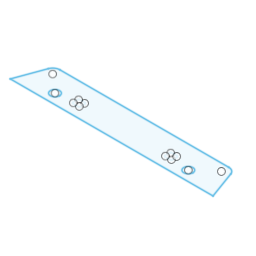
Zaagblad_C (Autodesk Fusion 360 archive; units mm, degrees)
design "Zaagblad_C" references "autodesk generic router xyz", "autodesk generic router xyz"
Autodesk Fusion 360 part; units mm, degrees
sketch "C_omtrek" plane through (0, 0, 0) normal (0, 0, 1) x (1, 0, 0)
  line L0 (0, -881.7664) -> (1220, -881.7664)
  line L1 (1220, -881.7664) -> (1220, -1491.7664)
  line L2 (1220, -1491.7664) -> (0, -1491.7664)
  line L3 (0, -1491.7664) -> (0, -881.7664)
  dimension "d47" = 610
  constraint horizontal L0
  constraint vertical L1
  constraint horizontal L2
  constraint vertical L3
  measures "d47" distance of L0.start L2.end
sketch "C_middle_holes" plane through (0, 0, 0) normal (0, 0, 1) x (1, 0, 0)
  line L0 (45, -1471.7664) -> (895, -1471.7664)
  line L1 (920, -1446.7664) -> (920, -926.7664)
  line L2 (895, -901.7664) -> (45, -901.7664)
  line L3 (20, -926.7664) -> (20, -1446.7664)
  arc A0 (20, -1446.7664) -> (45, -1471.7664) centre (45, -1446.7664) ccw
  arc A1 (45, -901.7664) -> (20, -926.7664) centre (45, -926.7664) ccw
  arc A2 (920, -926.7664) -> (895, -901.7664) centre (895, -926.7664) ccw
  arc A3 (895, -1471.7664) -> (920, -1446.7664) centre (895, -1446.7664) ccw
  line L4 (360, -1144.2664) -> (580, -1144.2664)
  line L5 (580, -1144.2664) -> (580, -1214.2664)
  line L6 (580, -1214.2664) -> (360, -1214.2664)
  line L7 (360, -1214.2664) -> (360, -1144.2664)
  line L8 (350, -1134.2664) -> (590, -1134.2664)
  line L9 (590, -1134.2664) -> (590, -1224.2664)
  line L10 (590, -1224.2664) -> (350, -1224.2664)
  line L11 (350, -1224.2664) -> (350, -1134.2664)
  circle A4 centre (280, -1179.2664) radius 48.25
  circle A5 centre (660, -1179.2664) radius 48.25
  line L12 (470, -1224.2664) -> (470, -1550) construction
  point P0 (20, -1471.7664)
  point P1 (920, -1471.7664)
  point P2 (20, -901.7664)
  dimension "d50" = 900
  dimension "d51" = 570
  dimension "d52" = 25
  dimension "d53" = 25
  dimension "d54" = 25
  dimension "d55" = 25
  dimension "d195" = -10
  dimension "d196" = 96.5
  dimension "d197" = 96.5
  constraint horizontal L0
  constraint vertical L1
  constraint horizontal L2
  constraint vertical L3
  constraint coincident P0 L0
  constraint coincident P0 L3
  constraint tangent L0 A0
  constraint tangent L3 A0
  constraint coincident P2 L2
  constraint coincident P2 L3
  constraint tangent L2 A1
  constraint tangent L3 A1
  constraint tangent L1 A2
  constraint tangent L2 A2
  constraint coincident P1 L0
  constraint coincident P1 L1
  constraint tangent L0 A3
  constraint tangent L1 A3
  constraint midpoint L10 L12.start
  constraint perpendicular L10 L12
  measures "d50" distance of P0 P1
  measures "d51" distance of P0 P2
  measures "d52" radius of A0
  measures "d53" radius of A1
  measures "d54" radius of A2
  measures "d55" radius of A3
  measures "d196" diameter of A4
  measures "d197" diameter of A5
extrude "Extrude1" add sketch "C_omtrek" along normal blind 18
sketch "C_bottom_edge" plane through (0, 0, 0) normal (0, 0, 1) x (1, 0, 0)
  line L0 (178.8438, -1361.7664) -> (743.8334, -1361.7664)
  line L1 (155.3514, -1378.2159) -> (121.3018, -1471.7664)
  arc A0 (178.8438, -1361.7664) -> (155.3514, -1378.2159) centre (178.8438, -1386.7664) ccw
  arc A1 (767.3257, -1378.2159) -> (743.8334, -1361.7664) centre (743.8334, -1386.7664) ccw
  line L2 (767.3257, -1378.2159) -> (801.3753, -1471.7664)
  line L3 (121.3018, -1471.7664) -> (801.3753, -1471.7664)
  dimension "d188" = 25
  dimension "d177" = 25
  dimension "d178" = 25
  constraint horizontal L0
  constraint tangent L1 A0
  constraint tangent L0 A0
  constraint tangent A1 L2
  constraint tangent L0 A1
  measures "d177" radius of A0
  measures "d178" radius of A1
sketch "C_bottom_holes" plane through (0, 0, 0) normal (0, 0, 1) x (1, 0, 0)
  circle A0 centre (246.75, -1438.2664) radius 15
  circle A1 centre (693.25, -1438.2664) radius 15
  line L0 (305.75, -1415.6268) -> (325.75, -1415.6268)
  line L1 (328.25, -1418.1268) -> (328.25, -1435.918)
  line L2 (325.75, -1438.418) -> (305.75, -1438.418)
  line L3 (303.25, -1435.918) -> (303.25, -1418.1268)
  arc A2 (328.25, -1418.1268) -> (325.75, -1415.6268) centre (325.75, -1418.1268) ccw
  arc A3 (305.75, -1415.6268) -> (303.25, -1418.1268) centre (305.75, -1418.1268) ccw
  arc A4 (303.25, -1435.918) -> (305.75, -1438.418) centre (305.75, -1435.918) ccw
  arc A5 (325.75, -1438.418) -> (328.25, -1435.918) centre (325.75, -1435.918) ccw
  arc A6 (634.25, -1438.418) -> (636.75, -1435.918) centre (634.25, -1435.918) ccw
  arc A7 (611.75, -1435.918) -> (614.25, -1438.418) centre (614.25, -1435.918) ccw
  arc A8 (636.75, -1418.1268) -> (634.25, -1415.6268) centre (634.25, -1418.1268) ccw
  arc A9 (614.25, -1415.6268) -> (611.75, -1418.1268) centre (614.25, -1418.1268) ccw
  line L4 (614.25, -1415.6268) -> (634.25, -1415.6268)
  line L5 (611.75, -1435.918) -> (611.75, -1418.1268)
  line L6 (634.25, -1438.418) -> (614.25, -1438.418)
  line L7 (636.75, -1418.1268) -> (636.75, -1435.918)
  point P0 (660, -1179.2664)
  point P1 (303.25, -1415.6268)
  point P2 (328.25, -1415.6268)
  point P3 (636.75, -1415.6268)
  point P4 (611.75, -1415.6268)
  dimension "d206" = 30
  dimension "d207" = 30
  dimension "d208" = 25
  dimension "d210" = 2.5
  dimension "d211" = 2.5
  dimension "d212" = 2.5
  dimension "d213" = 2.5
  dimension "d214" = 25
  dimension "d215" = 2.5
  dimension "d216" = 2.5
  dimension "d217" = 2.5
  dimension "d218" = 2.5
  constraint horizontal L0
  constraint vertical L1
  constraint horizontal L2
  constraint vertical L3
  constraint coincident P2 L0
  constraint coincident P2 L1
  constraint tangent L0 A2
  constraint tangent L1 A2
  constraint coincident P1 L0
  constraint coincident P1 L3
  constraint tangent L0 A3
  constraint tangent L3 A3
  constraint tangent L2 A4
  constraint tangent L3 A4
  constraint tangent L1 A5
  constraint tangent L2 A5
  constraint horizontal L4
  constraint vertical L7
  constraint horizontal L6
  constraint vertical L5
  constraint coincident P3 L4
  constraint coincident P3 L7
  constraint tangent A8 L4
  constraint tangent A8 L7
  constraint coincident P4 L4
  constraint coincident P4 L5
  constraint tangent A9 L4
  constraint tangent A9 L5
  constraint tangent A7 L6
  constraint tangent A7 L5
  constraint tangent A6 L7
  constraint tangent A6 L6
  measures "d206" diameter of A0
  measures "d207" diameter of A1
  measures "d208" distance of P1 P2
  measures "d210" radius of A2
  measures "d211" radius of A3
  measures "d212" radius of A4
  measures "d213" radius of A5
  measures "d214" distance of P3 P4
  measures "d215" radius of A8
  measures "d216" radius of A9
  measures "d217" radius of A7
  measures "d218" radius of A6
sketch "Lasercutter_3mm" plane through (0, 0, 0) normal (0, 0, 1) x (1, 0, 0)
  line L0 (580, -1144.2664) -> (580, -1214.2664)
  line L1 (895, -901.7664) -> (45, -901.7664)
  arc A0 (895, -1471.7664) -> (920, -1446.7664) centre (895, -1446.7664) ccw
  arc A1 (920, -926.7664) -> (895, -901.7664) centre (895, -926.7664) ccw
  circle A2 centre (660, -1179.2664) radius 48.25
  line L2 (360, -1144.2664) -> (580, -1144.2664)
  line L3 (920, -1446.7664) -> (920, -926.7664)
  line L4 (20, -926.7664) -> (20, -1446.7664)
  arc A3 (45, -901.7664) -> (20, -926.7664) centre (45, -926.7664) ccw
  line L5 (580, -1214.2664) -> (360, -1214.2664)
  arc A4 (20, -1446.7664) -> (45, -1471.7664) centre (45, -1446.7664) ccw
  circle A5 centre (280, -1179.2664) radius 48.25
  line L6 (360, -1214.2664) -> (360, -1144.2664)
  point P0 (660, -1179.2664)
  dimension "d219" = -10
  dimension "d222" = 25
  dimension "d223" = 25
  dimension "d224" = 25
  dimension "d225" = 25
  dimension "d226" = 96.5
  dimension "d227" = 96.5
  constraint vertical L3
  constraint horizontal L1
  constraint vertical L4
  constraint tangent L4 A4
  constraint tangent L1 A3
  constraint tangent L4 A3
  constraint tangent A1 L3
  constraint tangent L1 A1
  constraint tangent A0 L3
  measures "d222" radius of A4
  measures "d223" radius of A3
  measures "d224" radius of A1
  measures "d225" radius of A0
  measures "d226" diameter of A5
  measures "d227" diameter of A2
sketch "Lasercutter_5mm" plane through (0, 0, 0) normal (0, 0, 1) x (1, 0, 0)
  line L0 (636.75, -1418.1268) -> (636.75, -1435.918)
  line L1 (611.75, -1435.918) -> (611.75, -1418.1268)
  arc A0 (611.75, -1435.918) -> (614.25, -1438.418) centre (614.25, -1435.918) ccw
  arc A1 (614.25, -1415.6268) -> (611.75, -1418.1268) centre (614.25, -1418.1268) ccw
  line L2 (328.25, -1418.1268) -> (328.25, -1435.918)
  line L3 (303.25, -1435.918) -> (303.25, -1418.1268)
  arc A2 (303.25, -1435.918) -> (305.75, -1438.418) centre (305.75, -1435.918) ccw
  arc A3 (305.75, -1415.6268) -> (303.25, -1418.1268) centre (305.75, -1418.1268) ccw
  circle A4 centre (246.75, -1438.2664) radius 15
  arc A5 (636.75, -1418.1268) -> (634.25, -1415.6268) centre (634.25, -1418.1268) ccw
  line L4 (325.75, -1438.418) -> (305.75, -1438.418)
  arc A6 (634.25, -1438.418) -> (636.75, -1435.918) centre (634.25, -1435.918) ccw
  line L5 (614.25, -1415.6268) -> (634.25, -1415.6268)
  line L6 (130.4954, -1471.7664) -> (809.5046, -1471.7664)
  line L7 (634.25, -1438.418) -> (614.25, -1438.418)
  circle A7 centre (693.25, -1438.2664) radius 15
  arc A8 (328.25, -1418.1268) -> (325.75, -1415.6268) centre (325.75, -1418.1268) ccw
  arc A9 (325.75, -1438.418) -> (328.25, -1435.918) centre (325.75, -1435.918) ccw
  line L8 (305.75, -1415.6268) -> (325.75, -1415.6268)
  arc A10 (775.5173, -1378.3869) -> (752.4948, -1362.2664) centre (752.4948, -1386.7664) ccw
  line L9 (187.5052, -1362.2664) -> (752.4948, -1362.2664)
  arc A11 (187.5052, -1362.2664) -> (164.4827, -1378.3869) centre (187.5052, -1386.7664) ccw
  line L10 (164.4827, -1378.3869) -> (130.4954, -1471.7664)
  line L11 (775.5173, -1378.3869) -> (809.5046, -1471.7664)
  dimension "d252" = 30
  dimension "d253" = 30
  dimension "d255" = 2.5
  dimension "d256" = 2.5
  dimension "d257" = 2.5
  dimension "d258" = 2.5
  dimension "d260" = 2.5
  dimension "d261" = 2.5
  dimension "d262" = 2.5
  dimension "d263" = 2.5
  constraint horizontal L6
  constraint horizontal L8
  constraint vertical L2
  constraint horizontal L4
  constraint vertical L3
  constraint tangent A8 L8
  constraint tangent L2 A8
  constraint tangent A3 L8
  constraint tangent L3 A3
  constraint tangent A2 L4
  constraint tangent L3 A2
  constraint tangent L2 A9
  constraint tangent L4 A9
  constraint horizontal L5
  constraint vertical L0
  constraint horizontal L7
  constraint vertical L1
  constraint tangent A5 L5
  constraint tangent L0 A5
  constraint tangent A1 L5
  constraint tangent L1 A1
  constraint tangent A0 L7
  constraint tangent L1 A0
  constraint tangent L0 A6
  constraint tangent A6 L7
  constraint tangent A10 L11
  constraint tangent A10 L9
  constraint tangent A11 L10
  constraint tangent L9 A11
  measures "d252" diameter of A4
  measures "d253" diameter of A7
  measures "d255" radius of A8
  measures "d256" radius of A3
  measures "d257" radius of A2
  measures "d258" radius of A9
  measures "d260" radius of A5
  measures "d261" radius of A1
  measures "d262" radius of A0
  measures "d263" radius of A6
sketch "Sketch22" plane through (0, 0, 0) normal (0, 0, 1) x (1, 0, 0)
